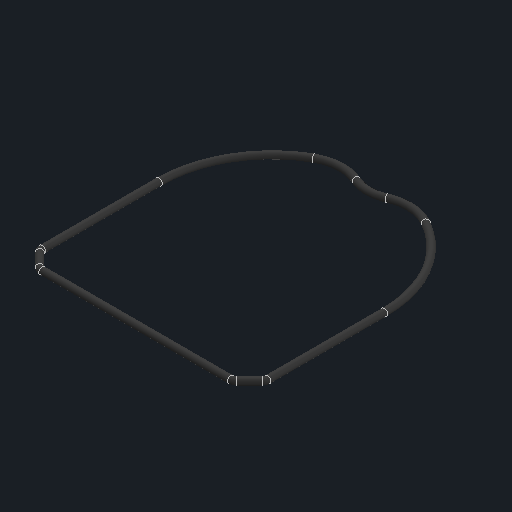
# Autodesk Inventor part: middle_gasket
Saved by Autodesk Inventor 2026.2 (Build 302298000, 298)
## iProperties
Created: 2026-04-07
Part Number: middle_gasket
Material: Rubber, Black
Document SubType Name: Modeling
Designer: Tathagata Sikdar
Density: 0.93 g/cm^3
Appearance: Rubber - Black
Author: Tathagata Sikdar
Autodesk Inventor part; units mm, degrees
ref_plane "YZ Plane" through (0, 0, 0) normal (1, 0, 0) x (0, 1, 0)
ref_plane "XZ Plane" through (0, 0, 0) normal (0, 1, 0) x (-1, 0, 0)
ref_plane "Work Plane1" through (60.2053, -12.7096, 92.2812) normal (0, 1, 0) x (-1, 0, 0)
sketch "Sketch1" plane through (60.2053, -12.7096, 92.2812) normal (0, 1, 0) x (-1, 0, 0)
  arc A0 (-40.6666, -82.6341) -> (-12.2349, -84.0587) centre (-25.049, -55.3704) ccw construction
  arc A1 (12.2349, -84.0587) -> (-12.2349, -84.0587) centre (0, -111.4504) ccw construction
  arc A2 (12.2349, -84.0587) -> (40.6666, -82.6341) centre (25.049, -55.3704) ccw construction
  arc A3 (40.6666, -82.6341) -> (81.8144, -11.6423) centre (0, -11.6423) ccw construction
  line L0 (81.8144, -11.6423) -> (81.8144, 75.1302) construction
  arc A4 (81.8144, 75.1302) -> (81.2286, 76.5444) centre (79.8144, 75.1302) ccw construction
  line L1 (81.2286, 76.5444) -> (71.5684, 86.2046) construction
  arc A5 (71.5684, 86.2046) -> (70.1542, 86.7904) centre (70.1542, 84.7904) ccw construction
  line L2 (70.1542, 86.7904) -> (-70.1542, 86.7904) construction
  arc A6 (-70.1542, 86.7904) -> (-71.5684, 86.2046) centre (-70.1542, 84.7904) ccw construction
  line L3 (-71.5684, 86.2046) -> (-81.2286, 76.5444) construction
  arc A7 (-81.2286, 76.5444) -> (-81.8144, 75.1302) centre (-79.8144, 75.1302) ccw construction
  line L4 (-81.8144, 75.1302) -> (-81.8144, -11.6423) construction
  arc A8 (-81.8144, -11.6423) -> (-40.6666, -82.6341) centre (0, -11.6423) ccw construction
  arc A9 (10, -81.3229) -> (-10, -81.3229) centre (0, -11.6423) ccw construction
  arc A10 (-39.9607, -81.4019) -> (-10, -81.3229) centre (-25.049, -55.3704) ccw construction
  arc A11 (-80.3944, -11.6423) -> (-39.9607, -81.4019) centre (0, -11.6423) ccw construction
  line L5 (-80.3944, 75.3704) -> (-80.3944, -11.6423) construction
  line L6 (-70.3944, 85.3704) -> (-80.3944, 75.3704) construction
  line L7 (70.3944, 85.3704) -> (-70.3944, 85.3704) construction
  line L8 (80.3944, 75.3704) -> (70.3944, 85.3704) construction
  line L9 (80.3944, -11.6423) -> (80.3944, 75.3704) construction
  arc A12 (39.9607, -81.4019) -> (80.3944, -11.6423) centre (0, -11.6423) ccw construction
  arc A13 (10, -81.3229) -> (39.9607, -81.4019) centre (25.049, -55.3704) ccw construction
  circle A14 centre (0, -11.6423) radius 68.3944 construction
  arc A15 (-87.3944, -11.6423) -> (87.3944, -11.6423) centre (0, -11.6423) ccw construction
  line L10 (87.3944, 88.3704) -> (87.3944, -11.6423) construction
  arc A16 (87.3944, 88.3704) -> (83.3944, 92.3704) centre (83.3944, 88.3704) ccw construction
  line L11 (-83.3944, 92.3704) -> (83.3944, 92.3704) construction
  arc A17 (-83.3944, 92.3704) -> (-87.3944, 88.3704) centre (-83.3944, 88.3704) ccw construction
  line L12 (-87.3944, -11.6423) -> (-87.3944, 88.3704) construction
  circle A18 centre (0, -95.5368) radius 1.85 construction
  circle A19 centre (-83.3944, 88.3704) radius 1.85 construction
  circle A20 centre (83.3944, 88.3704) radius 1.85 construction
  arc A21 (-85.9744, -11.6423) -> (-42.7343, -86.2438) centre (0, -11.6423) ccw construction
  line L13 (-85.9744, -11.6423) -> (-85.9744, 75.1302) construction
  arc A22 (-84.1702, 79.486) -> (-85.9744, 75.1302) centre (-79.8144, 75.1302) ccw construction
  line L14 (-84.1702, 79.486) -> (-74.51, 89.1462) construction
  arc A23 (-70.1542, 90.9504) -> (-74.51, 89.1462) centre (-70.1542, 84.7904) ccw construction
  line L15 (-70.1542, 90.9504) -> (70.1542, 90.9504) construction
  arc A24 (74.51, 89.1462) -> (70.1542, 90.9504) centre (70.1542, 84.7904) ccw construction
  line L16 (74.51, 89.1462) -> (84.1702, 79.486) construction
  arc A25 (85.9744, 75.1302) -> (84.1702, 79.486) centre (79.8144, 75.1302) ccw construction
  line L17 (85.9744, 75.1302) -> (85.9744, -11.6423) construction
  arc A26 (42.7343, -86.2438) -> (85.9744, -11.6423) centre (0, -11.6423) ccw construction
  arc A27 (10.5384, -87.857) -> (42.7343, -86.2438) centre (25.049, -55.3704) ccw construction
  arc A28 (10.5384, -87.857) -> (-10.5384, -87.857) centre (0, -111.4504) ccw construction
  arc A29 (-42.7343, -86.2438) -> (-10.5384, -87.857) centre (-25.049, -55.3704) ccw construction
  line L18 (-83.8944, -11.6423) -> (-83.8944, 75.1302)
  arc A30 (-82.6994, 78.0152) -> (-83.8944, 75.1302) centre (-79.8144, 75.1302) ccw
  line L19 (-82.6994, 78.0152) -> (-73.0392, 87.6754)
  arc A31 (-70.1542, 88.8704) -> (-73.0392, 87.6754) centre (-70.1542, 84.7904) ccw
  line L20 (-70.1542, 88.8704) -> (70.1542, 88.8704)
  arc A32 (73.0392, 87.6754) -> (70.1542, 88.8704) centre (70.1542, 84.7904) ccw
  line L21 (73.0392, 87.6754) -> (82.6994, 78.0152)
  arc A33 (83.8944, 75.1302) -> (82.6994, 78.0152) centre (79.8144, 75.1302) ccw
  line L22 (83.8944, 75.1302) -> (83.8944, -11.6423)
  arc A34 (41.7004, -84.439) -> (83.8944, -11.6423) centre (0, -11.6423) ccw
  arc A35 (11.3866, -85.9579) -> (41.7004, -84.439) centre (25.049, -55.3704) ccw
  arc A36 (11.3866, -85.9579) -> (-11.3866, -85.9579) centre (0, -111.4504) ccw
  arc A37 (-41.7004, -84.439) -> (-11.3866, -85.9579) centre (-25.049, -55.3704) ccw
  arc A38 (-83.8944, -11.6423) -> (-41.7004, -84.439) centre (0, -11.6423) ccw
  point P0 (60.2053, -92.2812)
  dimension "d0" = 2.08
  constraints: 18 point on circle, 10 end point, 9 centre point, 13 other
  measures "d0" distance between parallel lines of L18 L4
sketch "Sketch2" plane through (0, 0, 0) normal (1, 0, 0) x (0, 1, 0)
  circle A0 centre (-12.7096, 181.1516) radius 2.5
  point P0 (0, 0)
  dimension "d1" = 5
  constraints: 1 centre point, 1 coincident
  measures "d1" diameter of A0
sweep "Sweep1" add profiles "Sketch2" path "Sketch1"
body "Solid1"
